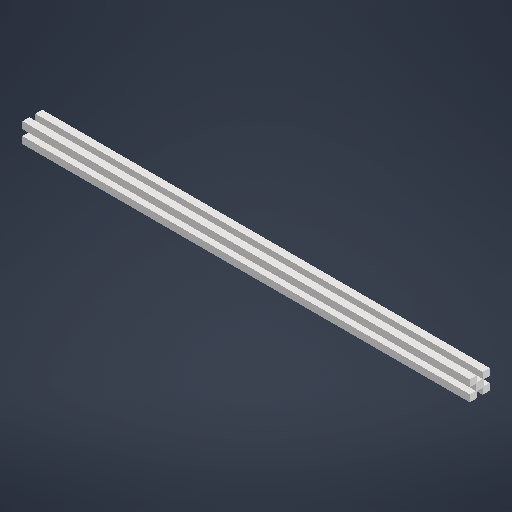
# Autodesk Inventor part: xbar
Saved by Autodesk Inventor 2025.1 (Build 291241020, 241B)
## iProperties
Created: 2024-09-23
Part Number: xbar
Material: Generic
Document SubType Name: Modeling
Designer: techn
Density: 1 g/cm^3
Appearance: Default
Author: techn
Autodesk Inventor part; units mm, degrees
ref_plane "YZ Plane" through (0, 0, 0) normal (1, 0, 0) x (0, 1, 0)
ref_plane "XZ Plane" through (0, 0, 0) normal (0, 1, 0) x (-1, 0, 0)
ref_plane "XY Plane" through (0, 0, 0) normal (0, 0, 1) x (1, 0, 0)
sketch "Sketch1" plane through (0, 0, 0) normal (0, 0, 1) x (1, 0, 0)
  line L0 (0, 0) -> (444, 0)
  line L1 (444, 0) -> (444, 3)
  line L2 (0, 3) -> (444, 3)
  line L3 (0, 0) -> (0, 3)
  line L4 (-3, 0) -> (-3, 3)
  line L5 (0, 3) -> (-3, 3)
  line L6 (0, 0) -> (-3, 0)
  line L7 (447, 0) -> (444, 0)
  line L8 (447, 0) -> (447, 3)
  line L9 (447, 3) -> (444, 3)
  line L10 (-3, -1.5) -> (447, -1.5)
  line L11 (-3, 4.5) -> (447, 4.5)
  line L12 (447, 4.5) -> (447, -1.5)
  line L13 (-3, -1.5) -> (-3, 4.5)
  line L14 (447, 4.5) -> (-3, 4.5)
  line L15 (-3, 4.5) -> (-3, 11.5)
  line L16 (-3, 11.5) -> (447, 11.5)
  line L17 (447, 11.5) -> (447, 4.5)
  line L18 (-3, -1.5) -> (447, -1.5)
  line L19 (447, -1.5) -> (447, -8.5)
  line L20 (447, -8.5) -> (-3, -8.5)
  line L21 (-3, -8.5) -> (-3, -1.5)
extrude "Extrusion1" add sketch "Sketch1" against normal blind 5 contours L10 L19 L20 L21 | L15 L16 L17 L11
sketch "Sketch3" plane through (0, 0, 0) normal (0, 0, 1) x (1, 0, 0)
  line L0 (-3, 4.5) -> (447, 4.5) projected
  line L1 (447, 4.5) -> (447, 11.5) projected
  line L2 (447, 11.5) -> (-3, 11.5) projected
  line L3 (-3, 11.5) -> (-3, 4.5) projected
  line L4 (0, 0) -> (444, 0) projected
  line L5 (444, 0) -> (444, 3) projected
  line L6 (0, 3) -> (444, 3) projected
  line L7 (0, 0) -> (0, 3) projected
  line L8 (447, -1.5) -> (-3, -1.5) projected
  line L9 (-3, -1.5) -> (-3, -8.5) projected
  line L10 (-3, -8.5) -> (447, -8.5) projected
  line L11 (447, -8.5) -> (447, -1.5) projected
  line L12 (-3, 0) -> (-3, 3) projected
  line L13 (0, 3) -> (-3, 3) projected
  line L14 (0, 0) -> (-3, 0) projected
  line L15 (447, 4.5) -> (447, -1.5) projected
  line L16 (447, 3) -> (444, 3) projected
  line L17 (447, 0) -> (444, 0) projected
  line L18 (444, 0) -> (444, 3) projected
  line L19 (-3, -1.5) -> (-3, 4.5) projected
extrude "Extrusion2" add sketch "Sketch3" along normal blind 1 contours L3 L2 L1 L0 | L8 L11 L10 L9
sketch "Sketch4" plane through (0, 0, 1) normal (0, 0, 1) x (1, 0, 0)
  line L0 (447, 4.5) -> (447, 11.5) projected
  line L1 (447, 11.5) -> (-3, 11.5) projected
  line L2 (-3, 11.5) -> (-3, 4.5) projected
  line L3 (-3, 4.5) -> (447, 4.5) projected
  line L4 (-3, -1.5) -> (-3, -8.5) projected
  line L5 (-3, -8.5) -> (447, -8.5) projected
  line L6 (447, -8.5) -> (447, -1.5) projected
  line L7 (447, -1.5) -> (-3, -1.5) projected
  line L8 (-3, 4.5) -> (-3, -1.5)
  line L9 (447, -1.5) -> (-3, -1.5) projected
  line L10 (447, 4.5) -> (447, -1.5)
  point P0 (0, 0)
  constraints: 4 end point, 1 perpendicular, 1 vertical
extrude "Extrusion3" add sketch "Sketch4" along normal blind 1
sketch "Sketch5" plane through (0, 0, 2) normal (0, 0, 1) x (1, 0, 0)
  line L0 (-3, 4.5) -> (447, 4.5) projected
  line L1 (-3, 4.5) -> (-3, -1.5) projected
  line L2 (447, -1.5) -> (-3, -1.5) projected
  line L3 (447, 11.5) -> (-3, 11.5) projected
  line L4 (-3, 11.5) -> (-3, -8.5) projected
  line L5 (-3, -8.5) -> (447, -8.5) projected
  line L6 (447, -8.5) -> (447, 11.5) projected
  line L7 (447, -2.5) -> (-4, -2.5)
  line L8 (-4, -2.5) -> (-4, 5.5)
  line L9 (-4, 5.5) -> (447, 5.5)
  line L10 (-3, -1.5) -> (-3, -2.5)
  line L11 (-3, 4.5) -> (-3, 5.5)
  line L12 (447, 11.5) -> (447, 4.5) projected
  line L13 (447, 5.5) -> (447, 4.5)
  line L14 (447, 4.5) -> (447, -2.5)
  point P0 (0, 0)
  point P1 (-3, -1.5)
  dimension "d12" = 1
  constraints: 14 end point, 4 point on line, 1 collinear, 1 vertical, 2 other
  measures "d12" distance between parallel lines of L2 L7
extrude "Extrusion4" add sketch "Sketch5" along normal blind 6 contours L4 L9 L6 L0 | L0 L6 L2 L1 | L2 L6 L7 L4
sketch "Sketch6" plane through (0, 0, 8) normal (0, 0, 1) x (1, 0, 0)
  line L0 (-3, 5.5) -> (447, 5.5) projected
  line L1 (447, 4.5) -> (-3, 4.5) projected
  line L2 (-3, 4.5) -> (-3, 11.5) projected
  line L3 (-3, 11.5) -> (447, 11.5) projected
  line L4 (447, 11.5) -> (447, 4.5) projected
  line L5 (-3, -1.5) -> (447, -1.5) projected
  line L6 (447, -1.5) -> (447, -8.5) projected
  line L7 (447, -8.5) -> (-3, -8.5) projected
  line L8 (-3, -8.5) -> (-3, -1.5) projected
  line L9 (-3, 5.5) -> (-3, -2.5) projected
  line L10 (-3, -2.5) -> (447, -2.5) projected
  line L11 (447, -2.5) -> (447, 5.5) projected
  line L12 (447, 5.5) -> (-3, 5.5) projected
  point P0 (0, 0)
extrude "Extrusion5" add sketch "Sketch6" along normal blind 1
sketch "Sketch7" plane through (0, 0, 9) normal (0, 0, 1) x (1, 0, 0)
  line L0 (-3, -1.5) -> (447, -1.5) projected
  line L1 (447, -1.5) -> (447, -8.5) projected
  line L2 (447, -8.5) -> (-3, -8.5) projected
  line L3 (-3, -8.5) -> (-3, -1.5) projected
  line L4 (447, 4.5) -> (-3, 4.5) projected
  line L5 (-3, 4.5) -> (-3, 11.5) projected
  line L6 (-3, 11.5) -> (447, 11.5) projected
  line L7 (447, 11.5) -> (447, 4.5) projected
  point P0 (0, 0)
extrude "Extrusion6" add sketch "Sketch7" along normal blind 6
body "Solid1"
